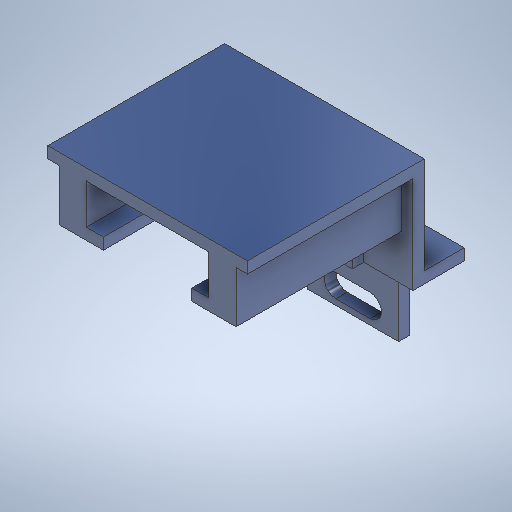
# Autodesk Inventor part: TapaCarcaza
Saved by Autodesk Inventor 2025.1 (Build 291241020, 241B)
## iProperties
Created: 2024-08-30
Part Number: TapaCarcaza
Material: Generic
Document SubType Name: Modeling
Designer: andre
Density: 1 g/cm^3
Appearance: Default
Author: andre
Autodesk Inventor part; units mm, degrees
ref_plane "YZ Plane" through (0, 0, 0) normal (1, 0, 0) x (0, 1, 0)
ref_plane "XZ Plane" through (0, 0, 0) normal (0, 1, 0) x (-1, 0, 0)
ref_plane "XY Plane" through (0, 0, 0) normal (0, 0, 1) x (1, 0, 0)
sketch "Sketch1" plane through (0, 0, 0) normal (0, 0, 1) x (1, 0, 0)
  line L0 (0, 0) -> (-5, 0)
  line L1 (-5, 0) -> (-5, 9)
  line L2 (-5, 9) -> (-9.75, 9)
  line L3 (-9.75, 9) -> (-9.75, 11)
  line L4 (-9.75, 11) -> (25.25, 11)
  line L5 (25.25, 11) -> (25.25, 9)
  line L6 (25.25, 9) -> (20.5, 9)
  line L7 (20.5, 9) -> (20.5, 0)
  line L8 (20.5, 0) -> (15.5, 0)
  line L9 (15.5, 0) -> (15.5, 2)
  line L10 (15.5, 2) -> (18.5, 2)
  line L11 (18.5, 2) -> (18.5, 9)
  line L12 (18.5, 9) -> (-3, 9)
  line L13 (-3, 9) -> (-3, 2)
  line L14 (-3, 2) -> (0, 2)
  line L15 (0, 0) -> (0, 2)
  dimension "d0" = 21.5
  dimension "d1" = 35
  dimension "d2" = 2
  dimension "d3" = 2
  dimension "d4" = 7
  dimension "d5" = 3
  dimension "d6" = 2
  constraints: 32 end point, 12 perpendicular, 6 point on line, 4 equal length, 1 coincident, 1 horizontal
  measures "d0" distance between parallel lines of L11 L13
  measures "d1" distance of L3.end L4.end
  measures "d2" distance between parallel lines of L13 L1
  measures "d3" distance between parallel lines of L0 L14
  measures "d4" distance between parallel lines of L12 L14
  measures "d5" distance of L13.end L14.end
  measures "d6" distance of L2.end L3.end
extrude "Extrusion1" add sketch "Sketch1" along normal blind 29
sketch "Sketch2" plane through (-9.75, 11, 0) normal (0, 1, 0) x (1, 0, 0)
  line L0 (0, 0) -> (4.75, 0) projected
  line L1 (0, 0) -> (35, 0)
  line L2 (35, 0) -> (35, 2)
  line L3 (35, 2) -> (0, 2)
  line L4 (0, 2) -> (0, 0)
  point P0 (9.75, 0)
  dimension "d9" = 2
  constraints: 8 end point, 2 parallel, 1 horizontal, 1 perpendicular, 1 vertical alignment
  measures "d9" distance between parallel lines of L1 L3
extrude "Extrusion2" add sketch "Sketch2" against normal blind 17
sketch "Sketch3" plane through (25.25, 11, -2) normal (0, 0, -1) x (-1, 0, 0)
  line L0 (10.6, -10) -> (19.6, -10)
  line L1 (19.6, -10) -> (19.6, -17)
  line L2 (19.6, -17) -> (10.6, -17)
  line L3 (10.6, -17) -> (10.6, -10)
  line L4 (35, -17) -> (0, -17) projected
  line L5 (0, 0) -> (0, -17) projected
  point P0 (25.25, -11)
  point P1 (15.1, -10)
  point P2 (17.5, -17)
  dimension "d13" = 9
  dimension "d26" = 10.6
  dimension "d53" = 7
  constraints: 8 end point, 2 midpoint, 2 parallel, 1 horizontal, 1 horizontal alignment, 1 perpendicular
  measures "d13" distance of L0.start L0.end
  measures "d26" distance between parallel lines of L5 L3
  measures "d53" distance of L2.end L0.start
extrude "Extrusion3" cut sketch "Sketch3" against normal blind 17
sketch "Sketch4" plane through (-3, 9, 0) normal (0, 0, 1) x (1, 0, 0)
  line L0 (17.65, -8) -> (17.65, -15) projected
  line L1 (28.25, -15) -> (17.65, -15) projected
  line L2 (28.25, 0) -> (28.25, -15) projected
  line L3 (23.5, 0) -> (28.25, 0) projected
  line L4 (23.5, -9) -> (23.5, 0) projected
  line L5 (18.5, -9) -> (23.5, -9) projected
  line L6 (18.5, -7) -> (18.5, -9) projected
  line L7 (21.5, -7) -> (18.5, -7) projected
  line L8 (21.5, 0) -> (21.5, -7) projected
  line L9 (0, 0) -> (21.5, 0) projected
  line L10 (0, -7) -> (0, 0) projected
  line L11 (3, -7) -> (0, -7) projected
  line L12 (3, -9) -> (3, -7) projected
  line L13 (-2, -9) -> (3, -9) projected
  line L14 (-2, 0) -> (-2, -9) projected
  line L15 (-6.75, 0) -> (-2, 0) projected
  line L16 (-6.75, 0) -> (-6.75, -15) projected
  line L17 (8.65, -15) -> (-6.75, -15) projected
  line L18 (8.65, -15) -> (8.65, -8) projected
  line L19 (8.65, -8) -> (17.65, -8) projected
  line L20 (19.65, -15) -> (19.65, -6)
  line L21 (19.65, -6) -> (6.65, -6)
  line L22 (6.65, -6) -> (6.65, -15)
  dimension "d16" = 2
  constraints: 6 end point, 2 point on line, 1 perpendicular, 2 other
  measures "d16" distance between parallel lines of L0 L20
extrude "Extrusion4" add sketch "Sketch4" along normal blind 2 and the other way blind 6.5 contours L19 L18 L17 L22 L21 L20 L7 L6 L5 L1 L0 | L5 L6 L7 L20
sketch "Sketch5" plane through (14.65, -6, -6.5) normal (-1, 0, 0) x (0, 0, 1)
  line L0 (8.5, 0) -> (0, 0) projected
  line L1 (0, 0) -> (8.5, 0)
  line L2 (8.5, 0) -> (8.5, -2)
  line L3 (8.5, -2) -> (0, -2)
  line L4 (0, -2) -> (0, 0)
  point P0 (6.5, 6)
  point P1 (8.5, 0)
  dimension "d21" = 2
  constraints: 8 end point, 2 parallel, 1 horizontal, 1 perpendicular
  measures "d21" distance of L1.end L2.end
extrude "Extrusion5" add sketch "Sketch5" along normal blind 12 and the other way blind 2
sketch "Sketch6" plane through (25.25, 11, -2) normal (0, 0, -1) x (-1, 0, 0)
  line L0 (0, 0) -> (0, -17) projected
  line L1 (0, -17) -> (35, -17)
  line L2 (35, -17) -> (35, -19)
  line L3 (35, -19) -> (0, -19)
  line L4 (0, -19) -> (0, -17)
  point P0 (25.25, -11)
  dimension "d27" = 2
  constraints: 8 end point, 2 parallel, 1 coincident, 1 horizontal, 1 perpendicular
  measures "d27" distance of L1.end L2.end
extrude "Extrusion6" add sketch "Sketch6" along normal blind 7 and the other way blind 2
sketch "Sketch7" plane through (2.65, -8, 2) normal (0, -1, 0) x (1, 0, 0)
  line L0 (14, 0) -> (14, -2) projected
  line L1 (14, 0) -> (0, 0) projected
  line L2 (0, -2) -> (0, 0) projected
  line L3 (-12.4, -2) -> (0, -2) projected
  line L4 (-12.4, -2) -> (-12.4, -11) projected
  line L5 (22.6, -11) -> (-12.4, -11) projected
  line L6 (22.6, -2) -> (22.6, -11) projected
  line L7 (14, -2) -> (22.6, -2) projected
  line L8 (22.6, -11) -> (-12.4, -11) projected
  line L9 (13.1, -11) -> (-2.9, -11)
  line L10 (-2.9, -11) -> (-2.9, -9)
  line L11 (-2.9, -9) -> (13.1, -9)
  line L12 (13.1, -9) -> (13.1, -11)
  point P0 (-2.65, -2)
  point P1 (5.1, -9)
  point P2 (5.1, -11)
  dimension "d32" = 16
  dimension "d33" = 2
  constraints: 8 end point, 2 midpoint, 2 parallel, 1 horizontal, 1 perpendicular, 1 point on line, 1 vertical alignment
  measures "d32" distance of L10.end L11.end
  measures "d33" distance of L11.end L9.start
extrude "Extrusion7" add sketch "Sketch7" along normal blind 16 contours L5 L10 L11 L12
sketch "Sketch8" plane through (25.25, 11, -9) normal (0, 0, -1) x (-1, 0, 0)
  arc A0 (14.5, -30) -> (14.5, -34) centre (14.5, -32) ccw
  arc A1 (20.5, -34) -> (20.5, -30) centre (20.5, -32) ccw
  line L0 (14.5, -30) -> (20.5, -30)
  line L1 (20.5, -34) -> (14.5, -34)
  line L2 (25.5, -35) -> (9.5, -35) projected
  point P0 (25.25, -11)
  point P1 (12.5, -32)
  point P2 (22.5, -32)
  point P3 (17.5, -34)
  point P4 (17.5, -30)
  point P5 (17.5, -35)
  point P6 (17.5, -35)
  dimension "d36" = 10
  dimension "d37" = 4
  dimension "d38" = 1
  constraints: 6 point on circle, 4 end point, 4 midpoint, 4 tangent, 2 centre point, 2 horizontal, 1 vertical alignment
  measures "d36" distance of point (12.5, -32) point (22.5, -32)
  measures "d37" distance of point (17.5, -34) point (17.5, -30)
  measures "d38" distance from line of point (17.5, -35) L1
extrude "Extrusion8" cut sketch "Sketch8" against normal blind 16
sketch "Sketch10" plane through (-3, 9, 0) normal (0, 0, 1) x (1, 0, 0)
  line L0 (21.5, -7) -> (19.65, -7) projected
  line L1 (21.5, 0) -> (21.5, -7) projected
  line L2 (0, 0) -> (21.5, 0) projected
  line L3 (0, -7) -> (0, 0) projected
  line L4 (3, -7) -> (0, -7) projected
  line L5 (3, -9) -> (3, -7) projected
  line L6 (-2, -9) -> (3, -9) projected
  line L7 (-2, 0) -> (-2, -9) projected
  line L8 (-6.75, 0) -> (-2, 0) projected
  line L9 (-6.75, 0) -> (-6.75, -17) projected
  line L10 (-6.75, -17) -> (5.65, -17) projected
  line L11 (6.65, -15) -> (6.65, -6) projected
  line L12 (-2, 0) -> (-4.75, 0)
  line L13 (-4.75, 0) -> (-4.75, -9)
  line L14 (-4.75, -9) -> (-2, -9)
  line L15 (-2, -9) -> (-2, 0)
  line L16 (23.5, -9) -> (23.5, 0) projected
  line L17 (23.5, 0) -> (26.25, 0)
  line L18 (26.25, 0) -> (26.25, -9)
  line L19 (26.25, -9) -> (23.5, -9)
  line L20 (23.5, -9) -> (23.5, 0)
  line L21 (28.25, 0) -> (28.25, -17) projected
  line L22 (19.65, -6) -> (19.65, -7) projected
  line L23 (5.65, -15) -> (5.65, -17) projected
  line L24 (6.65, -15) -> (5.65, -15) projected
  line L25 (6.65, -6) -> (19.65, -6) projected
  line L26 (19.65, -9) -> (19.65, -17) projected
  line L27 (19.65, -17) -> (28.25, -17) projected
  line L28 (28.25, 0) -> (28.25, -17) projected
  line L29 (23.5, 0) -> (28.25, 0) projected
  line L30 (23.5, -9) -> (23.5, 0) projected
  line L31 (19.65, -9) -> (23.5, -9) projected
  point P0 (18.5, -9)
  point P1 (-2, -9)
  point P2 (-4.75, 0)
  dimension "d44" = 2
  dimension "d45" = 2
  constraints: 16 end point, 4 parallel, 2 horizontal, 2 horizontal alignment, 2 perpendicular
  measures "d44" distance between parallel lines of L9 L13
  measures "d45" distance between parallel lines of L21 L18
extrude "Extrusion10" add sketch "Sketch10" along normal up to surface (29 mm away) contours L14 L13 L8 L7 | L16 L17 L18 L19
sketch "Sketch11" plane through (0, 0, 29) normal (0, 0, 1) x (1, 0, 0)
  line L0 (25.25, 11) -> (-9.75, 11) projected
  line L1 (0, 0) -> (-7.75, 0) projected
  line L2 (18.5, 9) -> (18.5, 2) projected
  line L3 (-3, 2) -> (-3, 9) projected
  line L4 (15.5, 2) -> (15.5, 0) projected
  line L5 (0, 0) -> (0, 2) projected
  point P0 (15.5, 1)
  point P1 (0, 1)
  dimension "d48" = 35
  dimension "d49" = 11
  dimension "d50" = 21.5
  dimension "d51" = 7
  dimension "d52" = 15.5
  constraints: 2 midpoint
  measures "d48" distance of L0.end L0.start
  measures "d49" distance between parallel lines of L0 L1
  measures "d50" distance between parallel lines of L2 L3
  measures "d51" distance of L3.start L3.end
  measures "d52" distance of point (15.5, 1) point (0, 1)
equation "\"d2\" = w"
equation "\"d3\" = w"
equation "\"d6\" = w"
equation "\"d9\" = w"
equation "\"d16\" = w"
equation "\"d33\" = w"
equation "\"d44\" = w"
equation "\"d45\" = w"
equation "\"w\" = 2"
body "Solid1"
